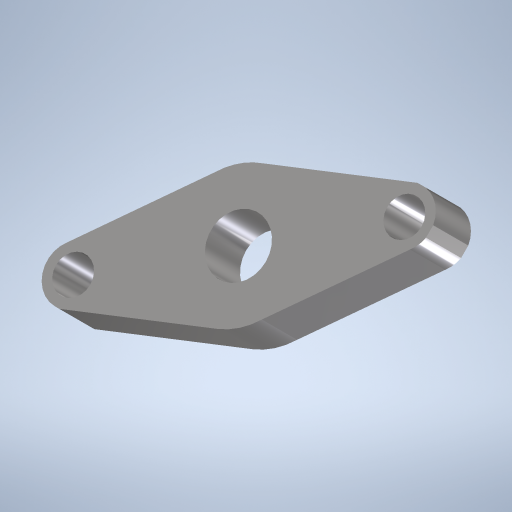
# Autodesk Inventor part: clamp_mechanism
Saved by Autodesk Inventor 2023 (Build 270158000, 158)
## iProperties
Created: 2023-11-21
Part Number: clamp_mechanism
Material: Steel, Mild
Document SubType Name: Modeling
Designer: Beatrice
Density: 7.85 g/cm^3
Appearance: Semi-Polished
Author: Beatrice
Autodesk Inventor part; units mm, degrees
ref_plane "YZ Plane" through (0, 0, 0) normal (1, 0, 0) x (0, 1, 0)
ref_plane "XZ Plane" through (0, 0, 0) normal (0, 1, 0) x (-1, 0, 0)
ref_plane "XY Plane" through (0, 0, 0) normal (0, 0, 1) x (1, 0, 0)
sketch "Sketch1" plane through (0, 0, 0) normal (1, 0, 0) x (0, 1, 0)
  circle A0 centre (-9.1612, 46.1081) radius 0.5 construction
  circle A1 centre (-9.1612, 46.1081) radius 0.9 construction
  line L0 (0, 43.0329) -> (-28.9151, 45.5627) construction
  line L1 (1.0918, 43.1767) -> (-27.4928, 38.1364) construction
  line L2 (-1.0918, 51.3262) -> (-28.367, 41.3989) construction
  line L3 (0, 51.4699) -> (-28.9151, 48.9402) construction
  line L4 (17.609, 51.9698) -> (-38.9081, 36.826) construction
  line L5 (18.2302, 47.2514) -> (-40.2807, 47.2514) construction
  line L6 (-2.4562, 42.2517) -> (-3.9425, 12.3724) construction
  line L7 (-19.1091, 33.3894) -> (19.1091, 33.3894) construction
  line L8 (-15.9499, 49.3393) -> (15.9499, 17.4395) construction
  line L9 (-15.9953, 17.3941) -> (15.9953, 49.3847) construction
  line L10 (2.4672, 42.2517) -> (3.9506, 12.3724) construction
  line L11 (-4.2099, 47.2514) -> (-6.25, 6.2414) construction
  line L12 (4.2215, 47.2514) -> (6.2448, 6.4952) construction
  circle A2 centre (-12.7187, 42.5506) radius 0.9 construction
  line L13 (-11.8457, 45.2351) -> (-10.9619, 46.119) construction
  line L14 (-10.9619, 46.119) -> (-9.1941, 44.3513) construction
  line L15 (-12.7296, 44.3513) -> (-13.501, 42.9956) construction
  line L16 (-11.8457, 45.2351) -> (-12.7296, 44.3513) construction
  line L17 (-10.9619, 42.5835) -> (-12.2433, 41.7864) construction
  line L18 (-12.7296, 44.3513) -> (-10.9619, 42.5835) construction
  line L19 (-10.9619, 46.119) -> (-9.6062, 46.8904) construction
  line L20 (-9.1941, 44.3513) -> (-10.078, 43.4674) construction
  line L21 (-10.9619, 42.5835) -> (-10.078, 43.4674) construction
  circle A3 centre (-12.7187, 42.5506) radius 0.5 construction
  line L22 (-13.4028, 41.8664) -> (-9.1612, 46.1081) construction
  line L23 (-9.1941, 44.3513) -> (-8.3969, 45.6327) construction
  line L24 (0.0006, 41.0008) -> (0, 41.0008) construction
  line L25 (0.0006, 41.0001) -> (0, 41.0001) construction
  line L26 (-2.4567, 42.2414) -> (2.4677, 42.2414) construction
  line L27 (2.4672, 42.2517) -> (-2.4562, 42.2517) construction
  line L28 (3, 47.2514) -> (4.2185, 47.2514) construction
  line L29 (0, 48.3894) -> (0, 48.3894) construction
  line L30 (-4.2185, 47.2514) -> (-4.2099, 47.2514) construction
  line L31 (0, 51.4699) -> (0, 43.0329) construction
  line L32 (-1.0918, 51.3262) -> (1.0918, 43.1767) construction
  ellipse E0 centre (0, 47.2514) end of major axis (-3, 47.2514) minor radius 3 (0.0225, 44.2515) -> (-0.0225, 44.2515) ccw construction
  circle A4 centre (0, 47.2514) radius 3 construction
  ellipse E1 centre (0, 47.2514) end of major axis (4.2185, 47.2514) minor radius 4.2127 (4.2185, 47.2514) -> (-4.2185, 47.2514) ccw construction
  circle A5 centre (0, 47.2514) radius 4.2185 construction
  line L33 (-6.0016, 11.2344) -> (6.0096, 11.2344) construction
  line L34 (-3.9425, 12.3724) -> (3.9506, 12.3724) construction
  ellipse E2 centre (0, 6.2414) end of major axis (-5, 6.2414) minor radius 5 construction
  ellipse E3 centre (0, 6.2414) end of major axis (6.25, 6.2414) minor radius 6.2414 (-6.2423, 6.5518) -> (6.2393, 6.6057) ccw construction
  line L35 (-28.1887, 40.7336) -> (-33.0183, 39.4395) construction
  line L36 (-34.1303, 30.7554) -> (-31, 33.8856) construction
  line L37 (-42.8892, 48.6033) -> (-22.6298, 28.3438) construction
  circle A6 centre (-31.7936, 38.7324) radius 0.2 construction
  circle A7 centre (-33.0183, 39.4395) radius 0.2 construction
  circle A8 centre (-32.7595, 38.4736) radius 0.6398 construction
  circle A9 centre (-32.7595, 38.4736) radius 0.6398 construction
  line L38 (-33.6434, 39.3574) -> (-31.8756, 37.5897) construction
  line L39 (-33.6434, 39.3574) -> (-31.5728, 39.3574) construction
  line L40 (-27.4928, 38.1364) -> (-28.367, 41.3989) construction
  line L41 (-28.9151, 45.5627) -> (-28.9151, 48.9402) construction
  line L42 (-34.0028, 47.2514) -> (-25.2783, 38.5269) construction
  line L43 (-28.1887, 40.7336) -> (-22.3931, 42.2865) construction
  line L44 (-21.5614, 39.1823) -> (-22.7073, 43.4588) construction
  line L45 (-27.6711, 38.8017) -> (-21.8755, 40.3546) construction
  line L46 (-32.5007, 37.5076) -> (-27.6711, 38.8017) construction
  line L47 (-42.7094, 48.4234) -> (-41.2248, 46.9389) construction
  line L48 (-33.0183, 39.4395) -> (-32.5007, 37.5076) construction
  circle A10 centre (-32.5007, 37.5076) radius 0.2 construction
  circle A11 centre (-32.7595, 38.4736) radius 1.01 construction
  circle A12 centre (-33.7254, 38.2147) radius 0.2 construction
  circle A13 centre (-32.7595, 38.4736) radius 1.25 construction
  line L49 (-31.8756, 37.5897) -> (-33.2898, 36.1755) construction
  line L50 (-31.8756, 37.5897) -> (-32.9109, 35.7965) construction
  line L51 (-35.0576, 37.9432) -> (-33.6434, 39.3574) construction
  line L52 (-32.9109, 35.7965) -> (-33.8666, 34.8408) construction
  line L53 (-33.2898, 36.1755) -> (-35.0576, 37.9432) construction
  line L54 (-35.4365, 38.3222) -> (-32.9109, 35.7965) construction
  line L55 (-36.3923, 37.3664) -> (-35.4365, 38.3222) construction
  line L56 (-33.8666, 34.8408) -> (-36.3923, 37.3664) construction
  line L57 (-31, 33.8856) -> (-41.6066, 44.4922) construction
  line L58 (-44.7369, 41.362) -> (-34.1303, 30.7554) construction
  line L59 (-43.1717, 42.9271) -> (-32.5651, 32.3205) construction
  line L60 (-33.6434, 39.3574) -> (-35.4365, 38.3222) construction
  circle A14 centre (-46.5116, 43.1367) radius 1.0497 construction
  line L61 (-47.1835, 40.9802) -> (-44.2042, 43.9595) construction
  line L62 (-46.1769, 46.993) -> (-47.2764, 45.8935) construction
  line L63 (-43.7409, 42.358) -> (-42.6414, 43.4574) construction
  line L64 (-43.1717, 42.9271) -> (-45.2366, 44.992) construction
  line L65 (-47.2764, 45.8935) -> (-43.7409, 42.358) construction
  line L66 (-45.8947, 42.269) -> (-42.5137, 45.6501) construction
  line L67 (-41.6066, 44.4922) -> (-44.7369, 41.362) construction
  line L68 (-48.6681, 42.4647) -> (-42.7094, 48.4234) construction
  line L69 (-41.9671, 47.6812) -> (-47.9258, 41.7225) construction
  line L70 (-41.2248, 46.9389) -> (-47.1835, 40.9802) construction
  line L71 (-42.6414, 43.4574) -> (-46.1769, 46.993) construction
  line L72 (-44.1236, 47.0092) -> (-42.6391, 45.5247) construction
  line L73 (-41.2248, 46.9389) -> (-44.2042, 43.9595) construction
  circle A15 centre (-43.3813, 46.2669) radius 1.0497 construction
  line L74 (-47.1835, 40.9802) -> (-48.6681, 42.4647) construction
  line L75 (-47.2538, 43.8789) -> (-45.7693, 42.3944) construction
  circle A16 centre (-43.3813, 46.2669) radius 1.0497 construction
  circle A17 centre (-46.5116, 43.1367) radius 1.05 construction
  circle A18 centre (-43.3813, 46.2669) radius 1.3 construction
  circle A19 centre (-46.5116, 43.1367) radius 1.3 construction
  line L76 (-41.9671, 47.6812) -> (-47.9258, 41.7225) construction
  line L77 (-47.9258, 41.7225) -> (-49.6936, 43.4902) construction
  line L78 (-49.6936, 43.4902) -> (-43.7349, 49.4489) construction
  line L79 (-43.7349, 49.4489) -> (-41.9671, 47.6812) construction
  line L80 (-41.9671, 47.6812) -> (-42.0968, 46.0669) construction
  line L81 (-47.9258, 41.7225) -> (-46.3116, 41.8522) construction
  line L82 (-44.9465, 44.7018) -> (-45.2271, 42.9367) construction
  line L83 (-44.9465, 44.7018) -> (-43.1813, 44.9824) construction
  line L84 (-44.801, 45.617) -> (-44.0639, 44.8421) construction
  line L85 (-44.0639, 44.8421) -> (-45.1697, 43.7902) construction
  line L86 (-45.1697, 43.7902) -> (-45.9068, 44.5651) construction
  line L87 (-45.9068, 44.5651) -> (-44.801, 45.617) construction
  line L88 (-44.801, 48.3828) -> (-49.0061, 44.1777) construction
  line L89 (-49.0061, 44.1777) -> (-52.5417, 47.7132) construction
  line L90 (-52.5417, 47.7132) -> (-48.3365, 51.9184) construction
  line L91 (-48.3365, 51.9184) -> (-44.801, 48.3828) construction
  line L92 (-46.9035, 50.4854) -> (-51.1087, 46.2803) construction
  line L93 (-44.801, 48.3828) -> (-43.7755, 47.3573)
  line L94 (-43.7755, 47.3573) -> (-47.9806, 43.1522)
  line L95 (-47.9806, 43.1522) -> (-49.0061, 44.1777)
  line L96 (-49.0061, 44.1777) -> (-44.801, 48.3828)
  line L97 (-46.1769, 46.993) -> (-45.1584, 45.9744)
  line L98 (-45.1584, 45.9744) -> (-46.2578, 44.875)
  line L99 (-46.2578, 44.875) -> (-47.2764, 45.8935)
  line L100 (-47.2764, 45.8935) -> (-46.1769, 46.993)
  point P0 (0, 0)
  point P1 (0, 0)
  point P2 (0, 33.3894)
  point P3 (-6.009, 41)
  point P4 (0, 47.2514)
  point P5 (0, 47.2514)
  point P6 (0, 0)
  point P7 (0, 0)
  point P8 (0, 12.3724)
  point P9 (0, 0)
  point P10 (28.7519, 36.3712)
  point P11 (-45.0774, 43.878)
  dimension "d12" = 3
  dimension "d13" = 5
  dimension "d14" = 6.2414
  dimension "d4" = 41.01
  dimension "d5" = 6.2414
  dimension "d6" = 4.993
  dimension "d7" = 5.69
  dimension "d8" = 29.869
  dimension "d9" = 1.138
  dimension "d10" = 2
  dimension "d11" = 90
  dimension "d15" = 15
  dimension "d16" = 2.5
  dimension "d17" = 1.25
  dimension "d18" = 60
  dimension "d19" = 2
  dimension "d20" = 1
  dimension "d21" = 6
  dimension "d22" = 1
  dimension "d23" = 1.8
  dimension "d24" = 5
  dimension "d25" = 2
  dimension "d26" = 2.02
  dimension "d27" = 2.5
  dimension "d28" = 0.4
  dimension "d29" = 360
  dimension "d30" = 150
  dimension "d31" = 15
  dimension "d32" = 15
  dimension "d33" = 5
  dimension "d34" = 0.75
  dimension "d35" = 4.2134
  dimension "d36" = 2
  dimension "d37" = 2.1
  dimension "d38" = 2.6
  dimension "d39" = 2.6
  dimension "d40" = 2.5
  dimension "d41" = 5
  dimension "d42" = 5.947
  constraints: 202 end point, 43 point on line, 29 parallel, 19 centre point, 19 perpendicular, 17 midpoint, 16 coincident, 11 symmetric about line, 10 point on circle, 4 collinear, 3 horizontal, 3 tangent, 2 horizontal alignment, 1 concentric, 1 equal length, 1 vertical alignment, 50 other
  measures "d4" distance of point (0, 47.251) point (0, 6.241)
  measures "d5" distance of point (0, 0) point (0, 6.241)
  measures "d6" distance from line of point (0, 6.241) L33
  measures "d7" angle of L11 L12
  measures "d8" distance between parallel lines of L34 L26
  measures "d9" distance between parallel lines of L33 L34
  measures "d10" distance between parallel lines of L11 L6
  measures "d11" angle of L8 L9
  measures "d16" distance between parallel lines of L16 L21
  measures "d17" distance between parallel lines of L8 L18
  measures "d18" angle of L42 L4
  measures "d19" distance between parallel lines of L45 L43
  measures "d20" distance between parallel lines of L43 L4
  measures "d21" distance between parallel lines of L44 L40
  measures "d22" diameter of A0
  measures "d23" diameter of A1
  measures "d24" distance between parallel lines of L48 L40
  measures "d25" distance of L38.end L49.end
  measures "d26" diameter of A11
  measures "d27" diameter of A13
  measures "d28" diameter of A7
  measures "d30" angle of L60 L39
  measures "d31" angle of L50 L49
  measures "d32" distance between parallel lines of L36 L67
  measures "d33" distance of L62.start L63.end
  measures "d34" distance between parallel lines of L71 L64
  measures "d35" distance from line of L61.end L37
  measures "d36" distance between parallel lines of L47 L72
  measures "d37" diameter of A17
  measures "d38" diameter of A18
  measures "d39" diameter of A19
  measures "d40" distance of L69.end L77.end
  measures "d41" distance between parallel lines of L78 L90
  measures "d42" distance between parallel lines of L91 L89
extrude "Extrusion1" add sketch "Sketch1" along normal mid plane 8
sketch "Sketch2" plane through (-4, -49.0061, 44.1777) normal (0, -0.7071068, 0.7071068) x (1, 0, 0)
  line L0 (0, 0) -> (8, 0) projected
  line L1 (8, 5.947) -> (8, 0) projected
  line L2 (8, 5.947) -> (0, 5.947) projected
  line L3 (0, 0) -> (0, 5.947) projected
  line L4 (0, 0) -> (8, 5.947)
  line L5 (0, 5.947) -> (0, 0) projected
  line L6 (0, 5.947) -> (8, 0)
  line L7 (0, 5.947) -> (8, 5.947) projected
  line L8 (4, 5.947) -> (4, -0.1076) construction
  line L9 (0, 2.9735) -> (8, 3) construction
  circle A0 centre (0.75, 0.75) radius 0.75
  circle A1 centre (4, 2.9735) radius 1.8
  line L10 (0.1438, 1.1916) -> (0.9981, 0.0422)
  circle A2 centre (0.7353, 5.2019) radius 0.75
  line L11 (0.1319, 4.7563) -> (0.9787, 5.9113)
  circle A3 centre (7.25, 0.75) radius 0.75
  line L12 (7.8562, 1.1916) -> (7.0019, 0.0422)
  line L13 (7.8681, 4.7563) -> (7.0213, 5.9113)
  circle A4 centre (7.2647, 5.2019) radius 0.75
  line L14 (2.6994, 4.2179) -> (0.1438, 1.1916)
  line L15 (0.8749, 0) -> (4.5834, 1.2707)
  line L16 (7.1253, 5.947) -> (3.4953, 4.7013)
  line L17 (7.8681, 4.7563) -> (5.295, 1.7233)
  line L18 (0, 5.947) -> (8, 5.947)
  line L19 (8, 5.947) -> (8, 0)
  line L20 (8, 0) -> (0, 0)
  line L21 (0, 0) -> (0, 5.947)
  circle A5 centre (4, 2.9735) radius 0.8
  circle A6 centre (0.75, 0.75) radius 0.5
  circle A7 centre (7.2647, 5.2019) radius 0.5
  point P0 (4, 3.4142)
  point P1 (8, 5.3499)
  point P2 (7.3505, 5.947)
  point P3 (8, 5.0539)
  point P4 (7.8027, 4.6793)
  point P5 (5.4446, 1.8996)
  point P6 (0, 0.75)
  point P7 (0.2132, 1.2737)
  point P8 (2.5554, 4.0474)
  point P9 (7.1253, 5.947)
  point P10 (0.75, 0)
  point P11 (4, 3)
  dimension "d45" = 1.5
  dimension "d46" = 3.6
  dimension "d49" = 1.6
  dimension "d52" = 1
  dimension "d53" = 1
  constraints: 32 end point, 12 point on circle, 9 symmetric about line, 8 centre point, 5 tangent, 4 coincident, 4 point on line, 3 midpoint, 2 parallel, 2 perpendicular, 1 horizontal, 1 vertical, 3 other
  measures "d45" diameter of A0
  measures "d46" diameter of A1
  measures "d49" diameter of A5
  measures "d52" diameter of A6
  measures "d53" diameter of A7
extrude "Extrusion2" cut sketch "Sketch2" against normal through all contours L4 A0 L0 | L3 A0 L4 | L3 A2 L6 L14 A0 | L15 A1 L6 A3 L0 | L3 A2 L6 L11 | A3 L6 L0 | A3 L12 L6 | L3 L6 A2 | L11 L6 A2 | L6 A2 L2 L16 A1 | L6 A3 L1 | A3 L6 L12 | L6 L12 A3 | L2 A2 L6 | A2 L2 L11 L6 | L6 L11 A2 | A3 L6 L17 A4 L1 | A3 L12 L6 | A4 L4 L1 | L4 A4 L2
extrude "Extrusion3" cut sketch "Sketch2" against normal through all contours A5 L4 L6 | L6 L4 A5 | L4 L6 A5 | L4 A5 L6
extrude "Extrusion4" cut sketch "Sketch2" against normal through all contours A6 L10 L4 | L4 L10 A6 | A6 L4 L10 | L4 A6 L10 | A7 L4 L13 | L13 L4 A7 | A7 L4 L13 | L13 L4 A7
body "Solid1"
